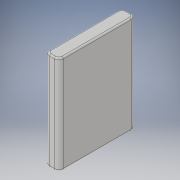
# Autodesk Inventor part: PKCell 3.7V 2500mAh
Saved by Autodesk Inventor 2018 (Build 220112000, 112)
## iProperties
Created: 2017-07-16
Part Number: PKCell 3.7V 2500mAh
Material: Generisch
Document SubType Name: Modeling
Designer: JochenAlt
Density: 1 g/cm^3
Appearance: Vorgabe
Author: JochenAlt
Autodesk Inventor part; units mm, degrees
ref_plane "YZ Plane" through (0, 0, 0) normal (1, 0, 0) x (0, 1, 0)
ref_plane "XZ Plane" through (0, 0, 0) normal (0, 1, 0) x (-1, 0, 0)
ref_plane "XY Plane" through (0, 0, 0) normal (0, 0, 1) x (1, 0, 0)
sketch "Skizze1" plane through (0, 0, 0) normal (1, 0, 0) x (0, 1, 0)
  line L0 (-25.5, -32.5) -> (25.5, -32.5)
  line L1 (25.5, -32.5) -> (25.5, 32.5)
  line L2 (25.5, 32.5) -> (-25.5, 32.5)
  line L3 (-25.5, 32.5) -> (-25.5, -32.5)
  line L4 (-25.5, -32.5) -> (25.5, 32.5) construction
  line L5 (25.5, -32.5) -> (-25.5, 32.5) construction
  point P0 (0, 0)
  dimension "d0" = 51
  dimension "d1" = 65
  constraints: 12 end point, 2 midpoint, 2 parallel, 1 horizontal, 1 perpendicular
  measures "d0" distance of L2.end L1.end
  measures "d1" distance of L1.end L0.end
extrude "Extrusion1" add sketch "Skizze1" along normal blind 9
fillet "Rundung1" radius 3 4 edges at (9, 25.5, 0) (0, 25.5, 0) (9, -25.5, 0) (0, -25.5, 0)
fillet "Rundung2" radius 1 16 edges at (8.1213, -24.6213, 32.5) (4.5, -25.5, 32.5) (0.8787, -24.6213, 32.5) (0, 0, 32.5) (0.8787, 24.6213, 32.5) (4.5, 25.5, 32.5) (8.1213, 24.6213, 32.5) (9, 0, 32.5) (8.1213, 24.6213, -32.5) (4.5, 25.5, -32.5) (0.8787, 24.6213, -32.5) (0, 0, -32.5) (0.8787, -24.6213, -32.5) (4.5, -25.5, -32.5) (8.1213, -24.6213, -32.5) (9, 0, -32.5)
sketch "Skizze2" plane through (0, 0, 0) normal (-1, 0, 0) x (0, 0, 1)
  circle A0 centre (0, 0) radius 5
  dimension "d6" = 10
  constraints: 1 centre point, 1 coincident
  measures "d6" diameter of A0
extrude "Extrusion2" add sketch "Skizze2" along normal blind 0.5
